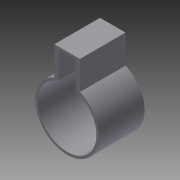
# Autodesk Inventor part: Neck
Saved by Autodesk Inventor 2015 (Build 190159000, 159)
## iProperties
Created: 2015-03-19
Part Number: Neck
Material: Generic
Document SubType Name: Modeling
Designer: ChristopherEvan
Density: 1 g/cm^3
Appearance: Default
Author: ChristopherEvan
Autodesk Inventor part; units mm, degrees
ref_plane "YZ Plane" through (0, 0, 0) normal (1, 0, 0) x (0, 1, 0)
ref_plane "XZ Plane" through (0, 0, 0) normal (0, 1, 0) x (-1, 0, 0)
ref_plane "XY Plane" through (0, 0, 0) normal (0, 0, 1) x (1, 0, 0)
ref_plane "Work Plane1" through (0, 0, 0) normal (0, 0, 1) x (1, 0, 0)
sketch "Sketch1" plane through (0, 0, 0) normal (0, 0, 1) x (1, 0, 0)
  line L0 (10.3879, -20.2759) -> (10.3879, 20.2759)
  line L1 (-9.35, -21.3138) -> (9.35, -21.3138)
  line L2 (-10.3879, -21.3138) -> (10.3879, -21.3138)
  line L3 (10.3879, -21.3138) -> (10.3879, 21.3138)
  line L4 (10.3879, 21.3138) -> (-10.3879, 21.3138)
  line L5 (-10.3879, 21.3138) -> (-10.3879, -21.3138)
  line L6 (-10.3879, -21.3138) -> (10.3879, 21.3138) construction
  line L7 (10.3879, -21.3138) -> (-10.3879, 21.3138) construction
  line L8 (-15.3879, 31.3138) -> (15.3879, 31.3138)
  arc A0 (-6.25, 26.7) -> (-3.75, 26.7) centre (-5, 24.8896) ccw projected
  arc A1 (3.75, 26.7) -> (6.25, 26.7) centre (5, 24.8896) ccw projected
  arc A2 (-3.75, -26.7) -> (-6.25, -26.7) centre (-5, -24.8896) ccw projected
  arc A3 (6.25, -26.7) -> (3.75, -26.7) centre (5, -24.8896) ccw projected
  circle A4 centre (-5, 24.8896) radius 2.2
  circle A5 centre (5, 24.8896) radius 2.2
  circle A6 centre (-5, -24.8896) radius 2.2
  circle A7 centre (5, -24.8896) radius 2.2
  circle A8 centre (0, -50.7404) radius 20.6245
  arc A9 (-15.3879, -3.1452) -> (15.3879, -3.1452) centre (0, -38.1663) ccw
  arc A10 (0.0421, 0.0864) -> (-0.0421, 0.0864) centre (0, -38.1663) ccw
  line L9 (15.3879, 31.3138) -> (15.3879, -3.1452)
  line L10 (-15.3879, -3.1452) -> (-15.3879, 31.3138)
  point P0 (0, 0)
  dimension "d0" = 10.3879
  dimension "d5" = 10
  constraints: 22 end point, 7 centre point, 4 coincident, 4 concentric, 4 point on circle, 2 midpoint, 2 point on line, 1 horizontal, 1 parallel, 1 perpendicular
  measures "d0" distance from line of L0 point (0, 0)
  measures "d5" distance between parallel lines of L4 L8
extrude "Extrusion1" add sketch "Sketch1" along normal blind 5
sketch "Sketch2" plane through (0, 0, 5) normal (0, 0, 1) x (1, 0, 0)
  arc A0 (-15.3879, -3.1452) -> (15.3879, -3.1452) centre (0, -38.1663) ccw projected
  arc A1 (-15.3879, -3.1452) -> (15.3879, -3.1452) centre (0, -38.1663) ccw
  circle A2 centre (-5, -24.8896) radius 2.2 projected
  circle A3 centre (5, -24.8896) radius 2.2 projected
  circle A4 centre (0, -50.7404) radius 20.6245 projected
  line L0 (-10.3879, -21.3138) -> (-10.3879, 21.3138) projected
  line L1 (10.3879, 21.3138) -> (10.3879, -21.3138) projected
  line L2 (10.3879, -21.3138) -> (-10.3879, -21.3138) projected
  line L3 (10.3879, -4.4789) -> (10.3879, -1.3511)
  line L4 (-10.3879, -1.3511) -> (-10.3879, -4.4789)
  line L5 (-15.3879, 31.3138) -> (15.3879, 31.3138)
  line L6 (15.3879, 31.3138) -> (15.3879, -3.1452)
  line L7 (-15.3879, -3.1452) -> (-15.3879, 31.3138)
  line L8 (10.3879, -4.4789) -> (10.3879, 21.3138)
  line L9 (-10.3879, 21.3138) -> (-10.3879, -4.4789)
  circle A5 centre (-5, 24.8896) radius 2.2 projected
  circle A6 centre (5, 24.8896) radius 2.2 projected
  circle A7 centre (0, -38.1663) radius 35.2526
  line L10 (10.3879, -4.4789) -> (10.3879, 28.3138)
  line L11 (10.3879, 28.3138) -> (-10.3879, 28.3138)
  line L12 (-10.3879, 28.3138) -> (-10.3879, -4.4789)
  point P0 (0, 0)
  dimension "d8" = 3
  dimension "d9" = 3
  constraints: 20 end point, 4 parallel, 4 point on circle, 2 centre point, 2 coincident, 1 concentric, 1 horizontal, 1 perpendicular
  measures "d8" distance between parallel lines of L5 L11
  measures "d9" radial gap between concentric circles of A0 A7
extrude "Extrusion2" add sketch "Sketch2" along normal blind 50 contours L7 L5 L6 A0
sketch "Sketch3" plane through (0, 0, 55) normal (0, 0, 1) x (1, 0, 0)
  line L0 (-15.3879, 31.3138) -> (-25.3879, 31.3138)
  line L1 (-25.3879, 31.3138) -> (-25.3879, 21.3138)
  line L2 (-25.3879, 21.3138) -> (-15.3879, 21.3138)
  line L3 (-15.3879, 31.3138) -> (-15.3879, -3.1452) projected
  line L4 (15.3879, 21.3138) -> (25.3879, 21.3138)
  line L5 (15.3879, -3.1452) -> (15.3879, 31.3138)
  line L6 (25.3879, 21.3138) -> (25.3879, 31.3138)
  line L7 (25.3879, 31.3138) -> (15.3879, 31.3138)
  arc A0 (-15.3879, -3.1452) -> (15.3879, -3.1452) centre (0, -38.1663) ccw projected
  line L8 (-25.3879, 31.3138) -> (-15.3879, 31.3138)
  line L9 (-15.3879, 31.3138) -> (-15.3879, 21.3138)
  line L10 (-15.3879, 21.3138) -> (-25.3879, 21.3138)
  line L11 (-25.3879, 21.3138) -> (-25.3879, 31.3138)
  line L12 (15.3879, 31.3138) -> (25.3879, 31.3138)
  line L13 (25.3879, 31.3138) -> (25.3879, 21.3138)
  line L14 (25.3879, 21.3138) -> (15.3879, 21.3138)
  line L15 (15.3879, 21.3138) -> (15.3879, 31.3138)
  circle A1 centre (-20.3879, 26.3138) radius 1
  circle A2 centre (20.3879, 26.3138) radius 1
  line L16 (-37.9245, -33.1663) -> (-48.2526, -33.1663)
  line L17 (-48.2526, -33.1663) -> (-48.2526, -43.1663)
  line L18 (-48.2526, -43.1663) -> (-37.9245, -43.1663)
  line L19 (-28.2526, -33.1663) -> (-48.2526, -43.1663) construction
  line L20 (-48.2526, -33.1663) -> (-28.2526, -43.1663) construction
  line L21 (-48.2526, -43.1663) -> (-38.2526, -43.1663)
  line L22 (-38.2526, -33.1663) -> (-48.2526, -33.1663)
  line L23 (-48.2526, -33.1663) -> (-48.2526, -43.1663)
  circle A3 centre (-43.2526, -38.1663) radius 1
  line L24 (48.2526, -33.1663) -> (37.9245, -33.1663)
  line L25 (37.9245, -43.1663) -> (48.2526, -43.1663)
  line L26 (48.2526, -43.1663) -> (48.2526, -33.1663)
  line L27 (48.2526, -33.1663) -> (28.2526, -43.1663) construction
  line L28 (28.2526, -33.1663) -> (48.2526, -43.1663) construction
  line L29 (48.2526, -43.1663) -> (38.2526, -43.1663)
  line L30 (38.2526, -33.1663) -> (48.2526, -33.1663)
  line L31 (48.2526, -33.1663) -> (48.2526, -43.1663)
  circle A4 centre (43.2526, -38.1663) radius 1
  circle A5 centre (0, -38.1663) radius 38.2526
  point P0 (0, 0)
  dimension "d14" = 20
  dimension "d15" = 10
  dimension "d16" = 2
  dimension "d18" = 10
  dimension "d19" = 2
  constraints: 62 end point, 10 horizontal, 8 parallel, 5 centre point, 4 point on circle, 3 perpendicular, 3 vertical, 2 point on line, 1 coincident, 13 other
  measures "d14" distance of L20.end L17.end
  measures "d15" distance of L17.end L16.end
  measures "d16" diameter of A3
  measures "d18" distance of L27.end L28.start
  measures "d19" diameter of A4
extrude "Extrusion4" add sketch "Sketch3" against normal blind 5 contours L3 L2 L1 L0 | L5 L7 L6 L4 | A0 L18 L17 L16 | L24 L26 L25 A0
body "Solid1"
